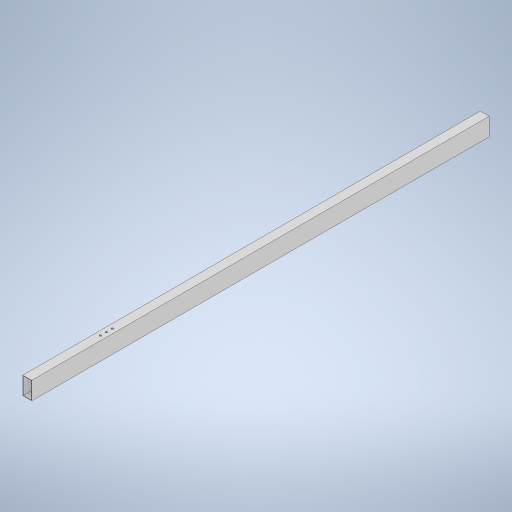
# Autodesk Inventor part: オムニ_角柱1_N
Saved by Autodesk Inventor 2023 (Build 270158000, 158)
## iProperties
Created: 2022-04-13
Part Number: オムニ_角柱1_N
Material: Generic
Document SubType Name: Sheet Metal
Designer: yuta
Density: 1 g/cm^3
Sheet Metal Rule: Default
Appearance: Default
Author: yuta
Autodesk Inventor part; units mm, degrees
ref_plane "YZ Plane" through (0, 0, 0) normal (1, 0, 0) x (0, 1, 0)
ref_plane "XZ Plane" through (0, 0, 0) normal (0, 1, 0) x (-1, 0, 0)
ref_plane "XY Plane" through (0, 0, 0) normal (0, 0, 1) x (1, 0, 0)
sketch "スケッチ1" plane through (0, 0, 0) normal (0, 0, 1) x (1, 0, 0)
  point P0 (0, 0)
sketch "スケッチ2" plane through (0, 0, 0) normal (0, 0, 1) x (1, 0, 0)
  line L0 (0, 0) -> (15, 0)
  line L1 (15, 0) -> (15, 30)
  line L2 (15, 30) -> (0, 30)
  line L3 (0, 30) -> (0, 0)
  dimension "d0" = 15
  dimension "d1" = 30
  constraints: 8 end point, 2 parallel, 1 horizontal, 1 perpendicular
  measures "d0" distance of L2.end L1.end
  measures "d1" distance of L1.end L0.end
extrude "押し出し1" add sketch "スケッチ2" along normal blind 770
sketch "スケッチ3" plane through (0, 0, 770) normal (0, 0, 1) x (1, 0, 0)
  line L0 (1, 1) -> (14, 1)
  line L1 (14, 1) -> (14, 29)
  line L2 (14, 29) -> (1, 29)
  line L3 (1, 29) -> (1, 1)
  line L4 (0, 30) -> (0, 0) projected
  line L5 (0, 0) -> (15, 0) projected
  dimension "d4" = 13
  dimension "d5" = 28
  dimension "d6" = 1
  dimension "d7" = 1
  constraints: 8 end point, 2 parallel, 1 horizontal, 1 perpendicular
  measures "d4" distance of L2.end L1.end
  measures "d5" distance of L1.end L0.end
  measures "d6" distance between parallel lines of L4 L3
  measures "d7" distance between parallel lines of L5 L0
extrude "押し出し2" cut sketch "スケッチ3" against normal blind 770
sketch "スケッチ4" plane through (0, 30, 770) normal (0, 1, 0) x (1, 0, 0)
  circle A0 centre (7.5, 123) radius 1.65
  line L0 (0, 770) -> (0, 0) projected
  line L1 (15, 0) -> (0, 0) projected
  circle A1 centre (7.5, 133) radius 1.65
  circle A2 centre (7.5, 143) radius 1.65
  dimension "d10" = 3.3
  dimension "d11" = 7.5
  dimension "d12" = 123
  dimension "d13" = 3.3
  dimension "d14" = 3.3
  dimension "d15" = 10
  dimension "d16" = 7.5
  dimension "d17" = 10
  dimension "d18" = 7.5
  constraints: 3 centre point
  measures "d10" diameter of A0
  measures "d11" distance from line of L0 A0.centre
  measures "d12" distance from line of L1 A0.centre
  measures "d13" diameter of A1
  measures "d14" diameter of A2
  measures "d15" distance of A0.centre A1.centre
  measures "d16" distance from line of L0 A1.centre
  measures "d17" distance of A1.centre A2.centre
  measures "d18" distance from line of L0 A2.centre
hole "穴1" at (7.5, 30, 647) at (7.5, 30, 637) at (7.5, 30, 627) direction (0, -1, 0) diameter 3.4 depth 30
equation "\"BendRadius\" = Thickness"
equation "\"BendReliefWidth\" = Thickness"
equation "\"BendReliefDepth\" = 0.5 * Thickness"
equation "\"CornerReliefSize\" = 4 * Thickness"
equation "\"MinimumRemnant\" = 2 * Thickness"
equation "\"TransitionRadius\" = BendRadius"
equation "\"JacobiRadiusSize\" = BendRadius"
equation "\"GapSize\" = Thickness"
equation "\"Thickness\" = 3.048"
